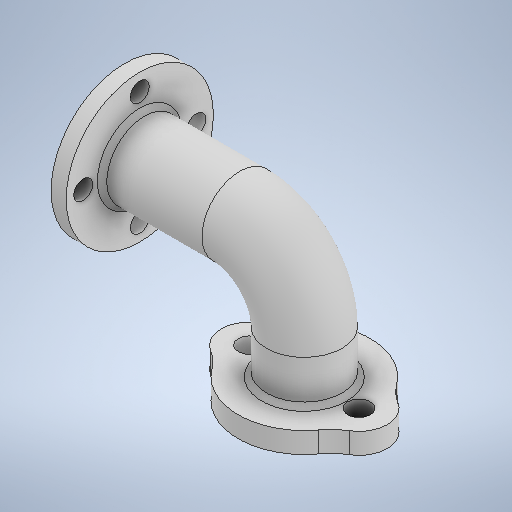
# Autodesk Inventor part: cad@41
Saved by Autodesk Inventor 2025.2 (Build 292293000, 293)
## iProperties
Created: 2025-03-30
Part Number: cad@41
Material: Generic
Document SubType Name: Modeling
Designer: spars
Density: 1 g/cm^3
Appearance: Default
Author: spars
Autodesk Inventor part; units mm, degrees
ref_plane "XZ Plane" through (0, 0, 0) normal (0, 1, 0) x (-1, 0, 0)
ref_plane "XY Plane" through (0, 0, 0) normal (0, 0, 1) x (1, 0, 0)
sketch "Sketch1" plane through (0, 0, 0) normal (0, 0, 1) x (1, 0, 0)
  line L0 (-244.3747, 73.9364) -> (-91.8552, 73.9364) construction
  line L1 (-91.8552, 73.9364) -> (-91.8552, -48.2612) construction
  line L2 (-91.8552, -48.2612) -> (-244.3747, -48.2612) construction
  line L3 (-244.3747, -48.2612) -> (-244.3747, 73.9364) construction
  line L4 (-19.331, 24.2448) -> (33.669, 24.2448)
  line L5 (68.669, -10.7552) -> (68.669, -33.7552)
  arc A0 (68.669, -10.7552) -> (33.669, 24.2448) centre (33.669, -10.7552) ccw
  point P0 (0, 0)
  dimension "d13" = 58
  dimension "d15" = 35
  constraints: 4 end point, 2 point on circle, 2 tangent, 1 centre point, 1 horizontal, 1 perpendicular, 2 other
  measures "d13" vertical distance of L5.end L4.start
  measures "d15" radius of A0
ref_plane "Work Plane1" through (-19.05, 0, 0) normal (1, 0, 0) x (0, 1, 0)
sketch "Sketch2" plane through (-19.05, 0, 0) normal (1, 0, 0) x (0, 1, 0)
  point P0 (0, 0)
sketch "Sketch3" plane through (-19.05, 0, 0) normal (1, 0, 0) x (0, 1, 0)
  circle A0 centre (23.454, 0) radius 20
  point P0 (0, 0)
  dimension "d16" = 40
  constraints: 1 centre point
  measures "d16" diameter of A0
sweep "Sweep1" add profiles "Sketch3" path "Sketch1"
shell "Shell1" thickness 7 removed faces 2 at (-19.331, 19.2276, 1.3227) at (61.9752, -33.7552, -3.0982)
sketch "Sketch4" plane through (-19.331, 23.454, 0) normal (-1, 0, 0) x (0, 0, 1)
  point P0 (0, -23.454)
sketch "Sketch5" plane through (-19.331, 23.454, 0) normal (-1, 0, 0) x (0, 0, 1)
  point P0 (0, -23.454)
sketch "Sketch6" plane through (-19.331, 23.454, 0) normal (-1, 0, 0) x (0, 0, 1)
  point P0 (0, -23.454)
sketch "Sketch7" plane through (-19.331, 23.454, 0) normal (-1, 0, 0) x (0, 0, 1)
  point P0 (0, -23.454)
sketch "Sketch8" plane through (-19.331, 23.454, 0) normal (-1, 0, 0) x (0, 0, 1)
  point P0 (0, -23.454)
sketch "Sketch9" plane through (-19.331, 23.454, 0) normal (-1, 0, 0) x (0, 0, 1)
  point P0 (0, -23.454)
sketch "Sketch10" plane through (-19.331, 23.454, 0) normal (-1, 0, 0) x (0, 0, 1)
  point P0 (0, -23.454)
sketch "Sketch11" plane through (-19.331, 23.454, 0) normal (-1, 0, 0) x (0, 0, 1)
  point P0 (0, -23.454)
sketch "Sketch12" plane through (-19.331, 23.454, 0) normal (-1, 0, 0) x (0, 0, 1)
  point P0 (0, -23.454)
sketch "Sketch13" plane through (-19.331, 23.454, 0) normal (-1, 0, 0) x (0, 0, 1)
  point P0 (0, -23.454)
sketch "Sketch14" plane through (-19.331, 23.454, 0) normal (-1, 0, 0) x (0, 0, 1)
  point P0 (0, -23.454)
sketch "Sketch15" plane through (-19.331, 23.454, 0) normal (-1, 0, 0) x (0, 0, 1)
  point P0 (0, -23.454)
sketch "Sketch16" plane through (-19.331, 23.454, 0) normal (-1, 0, 0) x (0, 0, 1)
  circle A0 centre (0, 0) radius 39
  circle A1 centre (0, 0) radius 13
  point P0 (0, -23.454)
  dimension "d20" = 78
  dimension "d21" = 26
  constraints: 2 centre point, 1 coincident
  measures "d20" diameter of A0
  measures "d21" diameter of A1
extrude "Extrusion1" add sketch "Sketch16" along normal blind 8
sketch "Sketch17" plane through (-27.331, 23.454, 0) normal (-1, 0, 0) x (0, 0, 1)
  circle A0 centre (0, 30) radius 5
  circle A1 centre (0, 0) radius 13 projected
  circle A2 centre (-30, 0) radius 5
  circle A3 centre (0, -30) radius 5
  circle A4 centre (30, 0) radius 5
  point P0 (0, -23.454)
  dimension "d24" = 10
  dimension "d25" = 30
  dimension "d28" = 360
  constraints: 4 centre point, 9 other
  measures "d24" diameter of A0
  measures "d25" distance of A1.centre A0.centre
extrude "Extrusion2" cut sketch "Sketch17" against normal blind 8 contours A0 | A2 | A3 | A4
chamfer "Chamfer1" distance 2.5 angle 45 1 edges at (-19.331, 3.454, 0)
sketch "Sketch18" plane through (67.8782, -33.7552, 0) normal (0, -1, 0) x (1, 0, 0)
  circle A0 centre (0, 0) radius 13 projected
  circle A1 centre (0, 0) radius 13
  circle A2 centre (29, 0) radius 6
  arc A3 (36.8103, -12.8062) -> (36.8103, 12.8062) centre (29, 0) ccw
  arc A4 (28.2321, 20.6869) -> (36.8103, 12.8062) centre (52.431, 38.4186) ccw
  arc A5 (36.8103, -12.8062) -> (28.2321, -20.6869) centre (52.431, -38.4186) ccw
  circle A6 centre (-29, 0) radius 6
  arc A7 (-36.8103, 12.8062) -> (-36.8103, -12.8062) centre (-29, 0) ccw
  arc A8 (-36.8103, 12.8062) -> (-28.2321, 20.6869) centre (-52.431, 38.4186) ccw
  arc A9 (-28.2321, -20.6869) -> (-36.8103, -12.8062) centre (-52.431, -38.4186) ccw
  arc A10 (28.2321, 20.6869) -> (-28.2321, 20.6869) centre (0, 0) ccw
  arc A11 (-28.2321, -20.6869) -> (28.2321, -20.6869) centre (0, 0) ccw
  point P0 (-67.8782, 0)
  dimension "d36" = 26
  dimension "d38" = 12
  dimension "d39" = 29
  dimension "d41" = 30
  dimension "d42" = 29
  constraints: 16 point on circle, 11 centre point, 4 coincident, 2 tangent, 1 equal radius
  measures "d36" diameter of A1
  measures "d38" diameter of A2
  measures "d39" distance of A0.centre A2.centre
  measures "d41" radius of A4
  measures "d42" distance of A6.centre A0.centre
extrude "Extrusion3" add sketch "Sketch18" along normal blind 11
chamfer "Chamfer2" distance 2.5 angle 45 1 edges at (47.8782, -33.7552, 0)
body "Solid1"
